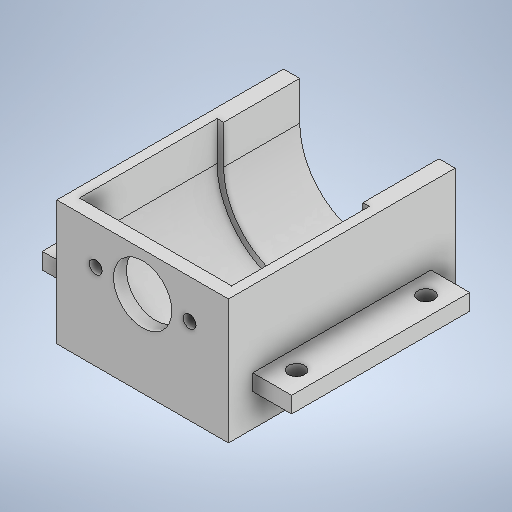
# Autodesk Inventor part: MotorCover
Saved by Autodesk Inventor 2025.3 (Build 293356000, 356)
## iProperties
Created: 2025-05-08
Part Number: MotorCover
Material: 일반
Document SubType Name: Modeling
Designer: 112-ROBOT-10
Density: 1 g/cm^3
Appearance: 기본값
Author: 112-ROBOT-10
## iProperties of the stored document MotorCover_3D 인쇄.ipt
Created: 2025-05-08
Part Number: MotorCover_3D 인쇄
Material: 일반
Document SubType Name: Modeling
Designer: SEON
Density: 1 g/cm^3
Appearance: 기본값
Author: SEON
Autodesk Inventor part; units mm, degrees
ref_plane "YZ Plane" through (0, 0, 0) normal (1, 0, 0) x (0, 1, 0)
ref_plane "XZ Plane" through (0, 0, 0) normal (0, 1, 0) x (-1, 0, 0)
sketch "스케치1" plane through (0, 0, 0) normal (0, 0, 1) x (1, 0, 0)
  line L0 (0, 0) -> (53, 0)
  line L1 (53, 0) -> (53, 38.5)
  line L2 (53, 38.5) -> (0, 38.5)
  line L3 (0, 38.5) -> (0, 0)
  arc A0 (3, 26.5) -> (6.2948, 38.5) centre (26.5, 26.5) ccw
  circle A1 centre (12, 26.5) radius 2
  circle A2 centre (41, 26.5) radius 2
  arc A3 (5, 26.5) -> (8.6604, 38.5) centre (26.5, 26.5) ccw
  circle A4 centre (26.5, 26.5) radius 9
  line L4 (3, 38.5) -> (3, 26.5)
  line L5 (5, 38.5) -> (5, 26.5)
  line L6 (48, 51.0228) -> (48, 26.5)
  line L7 (50, 50.0136) -> (50, 26.5)
  line L8 (26.5, 0) -> (26.5, 1.4842)
  line L9 (0, 28) -> (-15, 28)
  line L10 (-15, 28) -> (-15, 13)
  line L11 (-15, 13) -> (0, 13)
  circle A5 centre (-9, 20.5) radius 2.5
  line L12 (53, 28) -> (68, 28)
  line L13 (68, 28) -> (68, 13)
  line L14 (68, 13) -> (53, 13)
  circle A6 centre (62, 20.5) radius 2.5
  circle A7 centre (-9, 20.5) radius 5
  circle A8 centre (62, 20.5) radius 5
  point P0 (44.3396, 38.5)
  point P1 (8.6604, 38.5)
  point P2 (6.2948, 38.5)
  point P3 (46.7052, 38.5)
  point P4 (50, 38.5)
  point P5 (48, 38.5)
  point P6 (-15, 20.5)
  dimension "d1" = 47
  dimension "d2" = 3
  dimension "d3" = 3
  dimension "d4" = 3
  dimension "d5" = 4
  dimension "d6" = 29
  dimension "d7" = 14.5
  dimension "d8" = 10
  dimension "d9" = 43
  dimension "d16" = 18
  dimension "d23" = 15
  dimension "d24" = 15
  dimension "d25" = 6
  dimension "d26" = 5
  dimension "d27" = 13
  dimension "d30" = 10
  constraints: 30 end point, 9 centre point, 6 point on circle, 6 point on line, 6 symmetric about line, 5 vertical, 4 tangent, 3 coincident, 3 horizontal alignment, 3 perpendicular, 2 horizontal, 2 midpoint, 2 parallel, 1 equal radius, 2 other
  measures "d1" diameter of A0
  measures "d2" distance edge to line of A0 L0
  measures "d3" distance edge to line of A0 L1
  measures "d4" distance edge to line of A0 L3
  measures "d5" diameter of A1
  measures "d6" distance of A2.centre A1.centre
  measures "d7" distance of A0.centre A1.centre
  measures "d8" distance edge to line of A2 L2
  measures "d9" diameter of A3
  measures "d16" diameter of A4
  measures "d23" distance of L9.end L10.end
  measures "d24" distance of L9.start L9.end
  measures "d25" distance from line of L10 A5.centre
  measures "d26" diameter of A5
  measures "d27" distance between parallel lines of L0 L11
  measures "d30" diameter of A7
extrude "돌출1" add sketch "스케치1" along normal blind 4 contours L3 L2 L4 A0 L7 L1 L0 | L2 L5 A3 L6 A0 L4 | L2 A3 L5 | L7 A0 L6 L2 | L6 A0 L2 | A0 L6 A3 L2
extrude "돌출2" add sketch "스케치1" against normal blind 66 contours L3 L2 L4 A0 L7 L1 L0 | L2 L5 A3 L6 A0 L4 | L7 A0 L6 L2
extrude "돌출3" cut sketch "스케치1" against normal blind 42.5 contours L2 L5 A3 L6 A0 L4 | L2 A3 L5 | L7 A0 L6 L2 | L6 A0 L2 | A0 L6 A3 L2 | A1 | A2 | A4
ref_plane "작업 평면1" through (0, 10, 4) normal (0, -1, 0) x (1, 0, 0)
sketch "스케치2" plane through (0, 10, 4) normal (0, -1, 0) x (1, 0, 0)
  line L0 (0, -70) -> (0, 0) projected
  line L1 (0, 0) -> (0, -70) projected
  line L2 (0, 0) -> (53, 0) projected
  line L3 (53, 0) -> (0, 0) projected
  line L4 (10, 0) -> (14, 0) projected
  line L5 (39, 0) -> (43, 0) projected
  line L6 (17.5, 0) -> (35.5, 0) projected
  line L7 (53, -70) -> (53, 0) projected
  line L8 (53, -70) -> (53, 0) projected
  line L9 (0, -7.5) -> (-12, -7.5)
  line L10 (-12, -7.5) -> (-12, -62.5)
  line L11 (-12, -62.5) -> (0, -62.5)
  circle A0 centre (-6, -15) radius 2.5
  circle A1 centre (-6, -55) radius 2.5
  line L12 (26.5, 0) -> (26.5, -15)
  line L13 (53, -7.5) -> (65, -7.5)
  line L14 (65, -7.5) -> (65, -62.5)
  line L15 (65, -62.5) -> (53, -62.5)
  circle A2 centre (59, -15) radius 2.5
  circle A3 centre (59, -55) radius 2.5
  point P0 (0, -4)
  point P1 (-6, -62.5)
  point P2 (0, -35)
  point P3 (-12, -35)
  dimension "d36" = 5
  dimension "d37" = 5
  dimension "d39" = 55
  dimension "d40" = 12
  dimension "d41" = 40
  dimension "d42" = 20
  constraints: 14 end point, 6 symmetric about line, 4 centre point, 4 midpoint, 2 perpendicular, 2 point on line, 2 vertical alignment, 1 horizontal, 1 horizontal alignment, 1 parallel, 1 vertical, 2 other
  measures "d36" diameter of A0
  measures "d37" diameter of A1
  measures "d39" distance of L9.end L10.end
  measures "d40" distance between parallel lines of L0 L10
  measures "d41" distance of A0.centre A1.centre
  measures "d42" vertical distance of point (-12, -35) A0.centre
extrude "돌출6" add sketch "스케치2" against normal blind 5
equation "\"d7\" = 0.5 * d6"
equation "\"d42\" = 0.5 * d41"
